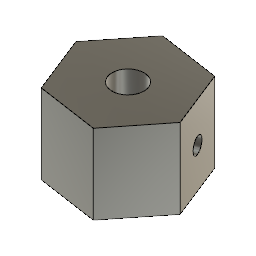
Wheel hub nut (Autodesk Fusion 360 design; units mm, degrees)
Autodesk Fusion 360 part; units mm, degrees
sketch "Sketch1" plane through (0, 0, 0) normal (0, 0, 1) x (1, 0, 0)
  line L0 (9.6196, 12.1538) -> (-5.7157, 14.4077)
  line L1 (-5.7157, 14.4077) -> (-15.3352, 2.2539)
  line L2 (-15.3352, 2.2539) -> (-9.6196, -12.1538)
  line L3 (-9.6196, -12.1538) -> (5.7157, -14.4077)
  line L4 (5.7157, -14.4077) -> (15.3352, -2.2539)
  line L5 (15.3352, -2.2539) -> (9.6196, 12.1538)
  circle A0 centre (0, 0) radius 4
  dimension "d2" = 15.5
  dimension "d4" = 8
  constraint coincident A0.centre origin
  measures "d2" distance of L0.start A0.centre
  measures "d4" diameter of A0
extrude "Extrude1" add sketch "Sketch1" along normal blind 20
sketch "Sketch2" plane through (12.4774, 4.9499, 0) normal (0.929527, 0.368753, 0) x (-0.368753, 0.929527, 0)
  line L0 (-7.75, 0) -> (7.75, 0)
  line L1 (7.75, 0) -> (7.75, 20)
  line L2 (7.75, 20) -> (-7.75, 20)
  line L3 (-7.75, 20) -> (-7.75, 0)
  circle A0 centre (0, 10) radius 2
  dimension "d10" = 4
  dimension "d11" = 10
  dimension "d12" = 7.75
  measures "d10" diameter of A0
  measures "d11" distance of L2 A0.centre
  measures "d12" distance of L1 A0.centre
extrude "Extrude2" cut sketch "Sketch2" against normal blind 115.5 contours A0
equation "hub_nut_polygon_radius = 7.75 mm"
equation "d2 = hub_nut_polygon_radius * 2"
equation "center_hole_radius = 4 mm"
equation "d4 = center_hole_radius * 2"
equation "thickness = 20 mm"
equation "extra = 100 mm"
equation "dowel_pin_hole_radius = 2 mm"
equation "d8 = thickness"
equation "d10 = dowel_pin_hole_radius * 2"
equation "d11 = thickness / 2"
equation "d12 = hub_nut_polygon_radius"
equation "d13 = -( hub_nut_polygon_radius * 2 + extra )"
